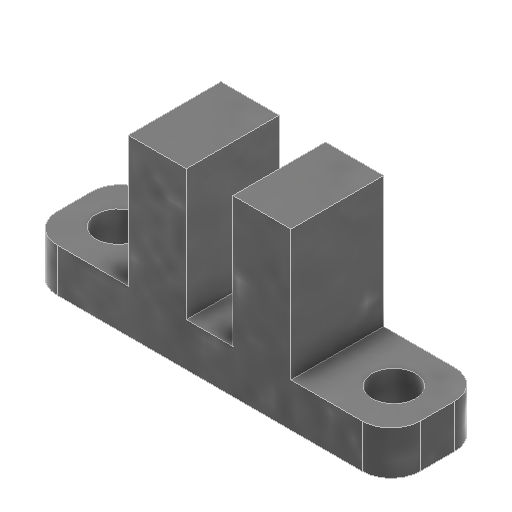
# Autodesk Inventor part: Sensor
Saved by Autodesk Inventor 2025.2 (Build 292293000, 293)
## iProperties
Created: 2025-05-05
Part Number: Sensor
Material: Generic
Document SubType Name: Modeling
Designer: nicoa
Density: 1 g/cm^3
Appearance: Fine Textured - Black
Author: nicoa
Autodesk Inventor part; units mm, degrees
ref_plane "YZ Plane" through (0, 0, 0) normal (1, 0, 0) x (0, 1, 0)
ref_plane "XZ Plane" through (0, 0, 0) normal (0, 1, 0) x (-1, 0, 0)
ref_plane "XY Plane" through (0, 0, 0) normal (0, 0, 1) x (1, 0, 0)
sketch "Sketch1" plane through (0, 0, 0) normal (0, 0, 1) x (1, 0, 0)
  line L0 (-12.5, -1.5) -> (12.5, -1.5)
  line L1 (12.5, -1.5) -> (12.5, 1.5)
  line L2 (12.5, 1.5) -> (-12.5, 1.5)
  line L3 (-12.5, 1.5) -> (-12.5, -1.5)
  line L4 (-12.5, -1.5) -> (12.5, 1.5) construction
  line L5 (12.5, -1.5) -> (-12.5, 1.5) construction
  line L6 (-5.6, 1.5) -> (-1.6, 1.5)
  line L7 (-1.6, 1.5) -> (-1.6, 10.5)
  line L8 (-1.6, 10.5) -> (-5.6, 10.5)
  line L9 (-5.6, 10.5) -> (-5.6, 1.5)
  line L10 (0, 1.5) -> (0, 12.2186)
  line L11 (1.6, 1.5) -> (1.6, 10.5)
  line L12 (1.6, 10.5) -> (5.6, 10.5)
  line L13 (5.6, 10.5) -> (5.6, 1.5)
  point P0 (0, 0)
  point P1 (5.6, 1.5)
  point P2 (1.6, 1.5)
  point P3 (-1.6, 1.5)
  dimension "d0" = 25
  dimension "d1" = 3
  dimension "d2" = 4
  dimension "d3" = 9
  dimension "d4" = 3.2
  constraints: 28 end point, 4 parallel, 4 symmetric about line, 3 midpoint, 2 horizontal, 2 perpendicular, 1 point on line, 1 vertical
  measures "d0" distance of L1.end L2.end
  measures "d1" distance of L0.end L1.end
  measures "d2" distance of L7.end L8.end
  measures "d3" distance of L6.end L7.end
  measures "d4" distance between parallel lines of L11 L7
extrude "Extrusion1" add sketch "Sketch1" along normal blind 6.38
sketch "Sketch2" plane through (5.6, 1.5, 0) normal (0, 1, 0) x (1, 0, 0)
  circle A0 centre (3.9, -3.19) radius 1.5
  line L0 (6.9, 0) -> (6.9, -6.38) projected
  circle A1 centre (-15.1, -3.19) radius 1.5
  line L1 (-18.1, 0) -> (-18.1, -6.38) projected
  point P0 (-5.6, 0)
  dimension "d7" = 3
  dimension "d8" = 3
  dimension "d9" = 3
  dimension "d10" = 3
  constraints: 2 centre point
  measures "d7" diameter of A0
  measures "d8" distance from line of L0 A0.centre
  measures "d9" diameter of A1
  measures "d10" distance from line of L1 A1.centre
extrude "Extrusion2" cut sketch "Sketch2" against normal through all
fillet "Fillet1" radius 2 4 edges at (12.5, 0, 6.38) (12.5, 0, 0) (-12.5, 0, 6.38) (-12.5, 0, 0)
body "Solid1"
